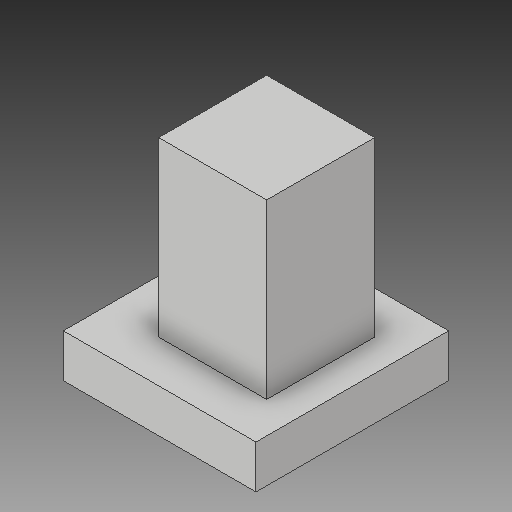
# Autodesk Inventor part: Stage 1 Plug
Saved by Autodesk Inventor 2018 (Build 220112000, 112)
## iProperties
Created: 2020-01-29
Part Number: Stage 1 Plug
Material: Generic
Document SubType Name: Modeling
Designer: 20quiletha
Density: 1 g/cm^3
Appearance: Default
Mass: 11.4944 g
Surface Area: 39.3641 cm^2
Volume: 11.4944 cm^3
Author: 20quiletha
Autodesk Inventor part; units mm, degrees
ref_plane "YZ Plane" through (0, 0, 0) normal (1, 0, 0) x (0, 1, 0)
ref_plane "XZ Plane" through (0, 0, 0) normal (0, 1, 0) x (-1, 0, 0)
ref_plane "XY Plane" through (0, 0, 0) normal (0, 0, 1) x (1, 0, 0)
sketch "Sketch1" plane through (0, 0, 0) normal (0, 1, 0) x (-1, 0, 0)
  line L0 (0, 0) -> (15.875, 0)
  line L1 (15.875, 0) -> (15.875, -15.875)
  line L2 (15.875, -15.875) -> (0, -15.875)
  line L3 (0, -15.875) -> (0, 0)
  dimension "d0" = 15.875
  dimension "d1" = 15.875
  constraints: 8 end point, 2 parallel, 1 horizontal, 1 perpendicular
  measures "d0" distance of L0.end L1.end
  measures "d1" distance of L1.end L2.end
extrude "Extrusion1" add sketch "Sketch1" along normal blind 25.4
sketch "Sketch3" plane through (0, 0, 0) normal (0, -1, 0) x (1, 0, 0)
  line L0 (-23.6855, -22.1107) -> (4.6355, -22.1107)
  line L1 (4.6355, -22.1107) -> (4.6355, 6.2103)
  line L2 (4.6355, 6.2103) -> (-23.6855, 6.2103)
  line L3 (-23.6855, 6.2103) -> (-23.6855, -22.1107)
  line L4 (-23.6855, -22.1107) -> (4.6355, 6.2103) construction
  line L5 (4.6355, -22.1107) -> (-23.6855, 6.2103) construction
  line L6 (0, 0) -> (-15.875, 0) projected
  line L7 (0, -15.875) -> (0, 0) projected
  line L8 (-15.875, 0) -> (-15.875, -15.875) projected
  point P0 (-9.525, -7.9502)
  dimension "d15" = 28.321
  dimension "d16" = 28.321
  dimension "d17" = 7.9502
  dimension "d21" = 6.35
  constraints: 12 end point, 2 midpoint, 2 parallel, 1 horizontal, 1 perpendicular
  measures "d15" distance of L1.end L2.end
  measures "d16" distance of L2.end L0.start
  measures "d17" distance from line of L6 point (-9.525, -7.95)
  measures "d21" distance from line of L8 point (-9.525, -7.95)
extrude "Extrusion3" add sketch "Sketch3" along normal blind 6.35
equation "\"d16\" = d15"
body "Solid1"
